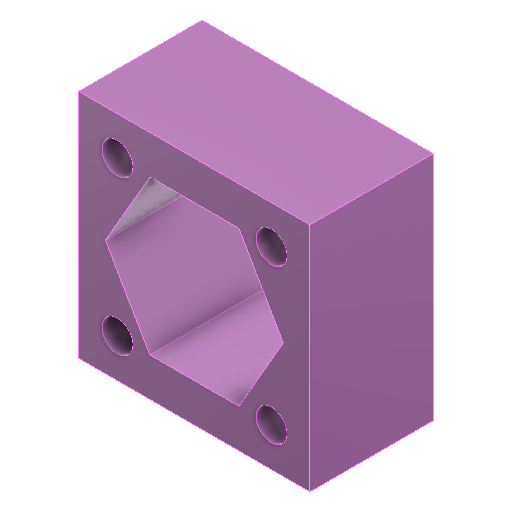
# Autodesk Inventor part: sujecion_cable
Saved by Autodesk Inventor 2026.1 (Build 301233000, 233)
## iProperties
Created: 2025-10-01
Part Number: sujecion_cable
Material: Genérico
Document SubType Name: Modeling
Designer: gianm
Density: 1 g/cm^3
Appearance: Suave - Púrpura
Author: gianm
Autodesk Inventor part; units mm, degrees
ref_plane "YZ Plane" through (0, 0, 0) normal (1, 0, 0) x (0, 1, 0)
ref_plane "XZ Plane" through (0, 0, 0) normal (0, 1, 0) x (-1, 0, 0)
ref_plane "XY Plane" through (0, 0, 0) normal (0, 0, 1) x (1, 0, 0)
sketch "Boceto1" plane through (0, 0, 0) normal (0, 0, 1) x (1, 0, 0)
  circle A0 centre (0, 0) radius 3
  line L0 (-2.8868, 5) -> (2.8868, 5)
  line L1 (2.8868, 5) -> (5.7735, 0)
  line L2 (5.7735, 0) -> (2.8868, -5)
  line L3 (2.8868, -5) -> (-2.8868, -5)
  line L4 (-2.8868, -5) -> (-5.7735, 0)
  line L5 (-5.7735, 0) -> (-2.8868, 5)
  line L6 (-7.5, -7.5) -> (7.5, -7.5)
  line L7 (7.5, -7.5) -> (7.5, 7.5)
  line L8 (7.5, 7.5) -> (-7.5, 7.5)
  line L9 (-7.5, 7.5) -> (-7.5, -7.5)
  line L10 (-7.5, -7.5) -> (7.5, 7.5) construction
  line L11 (7.5, -7.5) -> (-7.5, 7.5) construction
  dimension "d0" = 6
  dimension "d1" = 10
  dimension "d2" = 15
  constraints: 24 end point, 2 coincident, 2 horizontal, 2 midpoint, 2 parallel, 2 perpendicular, 1 centre point, 13 other
  measures "d0" diameter of A0
  measures "d1" distance between parallel lines of L0 L3
  measures "d2" distance of L7.end L8.end
extrude "Extrusión1" add sketch "Boceto1" against normal blind 8 contours L9 L8 L7 L6
sketch "Boceto2" plane through (0, 0, -8) normal (0, 0, -1) x (-1, 0, 0)
  circle A0 centre (-5, 5) radius 1
  line L0 (5, -5) -> (-5, -5) construction
  line L1 (-5, -5) -> (-5, 5) construction
  line L2 (-5, 5) -> (5, 5) construction
  line L3 (5, 5) -> (5, -5) construction
  line L4 (5, -5) -> (-5, 5) construction
  line L5 (-5, -5) -> (5, 5) construction
  circle A1 centre (5, 5) radius 1
  circle A2 centre (5, -5) radius 1
  circle A3 centre (-5, -5) radius 1
  point P0 (0, 0)
  dimension "d5" = 10
  dimension "d6" = 2
  constraints: 12 end point, 4 centre point, 3 coincident, 3 equal radius, 2 midpoint, 2 parallel, 2 perpendicular, 1 horizontal
  measures "d5" distance of L1.end L2.end
  measures "d6" diameter of A1
extrude "Extrusión2" cut sketch "Boceto2" against normal up to surface (8 mm away)
